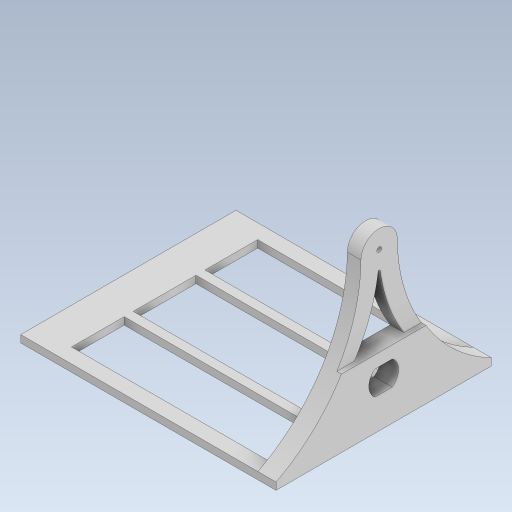
# Autodesk Inventor part: base plate main
Saved by Autodesk Inventor 2023 (Build 270158000, 158)
## iProperties
Created: 2023-03-24
Part Number: base plate main
Material: Generic
Document SubType Name: Modeling
Designer: AggyT
Density: 1 g/cm^3
Appearance: Default
Author: AggyT
Autodesk Inventor part; units mm, degrees
ref_plane "YZ Plane" through (0, 0, 0) normal (1, 0, 0) x (0, 1, 0)
ref_plane "XZ Plane" through (0, 0, 0) normal (0, 1, 0) x (-1, 0, 0)
sketch "Sketch1" plane through (0, 0, 0) normal (0, 1, 0) x (-1, 0, 0)
  line L0 (0, 0) -> (-203.2, 0)
  line L1 (-203.2, 0) -> (-203.2, -177.8)
  line L2 (-203.2, -177.8) -> (0, -177.8)
  line L3 (0, -177.8) -> (0, 0)
  dimension "d0" = 203.2
  dimension "d1" = 177.8
  constraints: 8 end point, 2 parallel, 1 horizontal, 1 perpendicular
  measures "d0" distance of L2.end L1.end
  measures "d1" distance of L1.end L0.end
extrude "Extrusion1" add sketch "Sketch1" along normal blind 10.16
sketch "Sketch2" plane through (0, 10.16, 0) normal (0, 1, 0) x (1, 0, 0)
  line L0 (203.2, 0) -> (203.2, 177.8) projected
  line L1 (203.2, 0) -> (177.8, 0)
  line L2 (177.8, 0) -> (177.8, 177.8)
  line L3 (177.8, 177.8) -> (203.2, 177.8)
  line L4 (203.2, 177.8) -> (203.2, 0)
  point P0 (0, 0)
  dimension "d4" = 25.4
  constraints: 8 end point, 2 parallel, 1 horizontal, 1 perpendicular
  measures "d4" distance of L2.end L3.end
extrude "Extrusion2" add sketch "Sketch2" along normal blind 42.5408
sketch "Sketch3" plane through (177.8, 10.16, -177.8) normal (-1, 0, 0) x (0, 0, 1)
  circle A0 centre (88.9, 25.4) radius 10.3886
  line L0 (81.407, 32.5957) -> (96.393, 32.5957)
  line L1 (81.5172, 18.0912) -> (96.2828, 18.0912)
  line L2 (0, 0) -> (177.8, 0) projected
  line L3 (82.9273, 33.9) -> (94.8727, 33.9)
  line L4 (82.9273, 16.9) -> (94.8727, 16.9)
  point P0 (177.8, -10.16)
  point P1 (88.9, -101.6)
  point P2 (88.8996, -101.6)
  point P3 (100.9466, -114.2832)
  point P4 (102.2534, -114.2832)
  point P5 (114.3004, -101.6)
  point P6 (114.3, -101.6)
  point P7 (159.1068, 0)
  point P8 (88.9, -76.6381)
  point P9 (114.2997, -101.509)
  point P10 (18.6932, 0)
  dimension "d7" = 20.7772
  dimension "d9" = 14.986
  dimension "d45" = 25.4
  dimension "d58" = 8.5
  dimension "d59" = 8.5
  constraints: 8 end point, 2 horizontal, 2 parallel, 10 other
  measures "d9" distance of L0.start L0.end
  measures "d45" distance from line of L2 point (88.9, 25.4)
  measures "d58" distance from line of point (88.9, 25.4) L3
  measures "d59" distance from line of L4 point (88.9, 25.4)
extrude "Extrusion3" cut sketch "Sketch3" against normal blind 50.8 contours A0 L1 L0
sketch "Sketch5" plane through (177.8, 10.16, -177.8) normal (-1, 0, 0) x (0, 0, 1)
  line L0 (-12.7, 203.2) -> (190.5, 203.2)
  line L1 (190.5, 203.2) -> (190.5, 0)
  line L2 (-12.7, 0) -> (-12.7, 203.2)
  line L3 (-12.7, 101.6) -> (190.5, 101.6)
  circle A0 centre (88.9, 101.6) radius 1.5635
  circle A1 centre (88.9, 101.6) radius 12.7
  arc A2 (13.581, 0) -> (76.2003, 101.691) centre (-39.021, 102.5166) ccw
  arc A3 (23.8054, 0) -> (88.9, 95.25) centre (-25.9987, 103.9047) ccw
  line L4 (88.9, -246.9942) -> (88.9, 203.2)
  arc A4 (101.5997, 101.691) -> (164.219, 0) centre (216.821, 102.5166) ccw
  arc A5 (88.9, 95.25) -> (153.9946, 0) centre (203.7987, 103.9047) ccw
  line L5 (153.9946, 0) -> (164.219, 0)
  line L6 (13.581, 0) -> (23.8054, 0)
  line L7 (-12.7, 0) -> (190.5, 0)
  line L8 (177.8, 0) -> (0, 0) projected
  line L9 (177.8, 42.5408) -> (0, 42.5408) projected
  line L10 (88.9, 42.5408) -> (88.9, 0)
  line L11 (0, 0) -> (177.8, 0) projected
  line L12 (13.581, 0) -> (-12.7, 0)
  line L13 (164.219, 0) -> (190.5, 0)
  point P0 (177.8, -10.16)
  point P1 (88.9, -101.6)
  point P2 (88.8996, -101.6)
  point P3 (100.9466, -114.2832)
  point P4 (102.2534, -114.2832)
  point P5 (114.3004, -101.6)
  point P6 (114.3, -101.6)
  point P7 (159.1068, 0)
  point P8 (88.9, -21.8971)
  point P9 (114.2997, -101.509)
  point P10 (88.9, 0)
  point P11 (76.2, 101.6)
  point P12 (76.1996, 101.6)
  point P13 (59.3636, 42.5408)
  point P14 (71.5262, 42.5408)
  point P15 (88.2466, 88.9168)
  point P16 (89.5534, 88.9168)
  point P17 (106.2738, 42.5408)
  point P18 (118.4364, 42.5408)
  point P19 (101.6004, 101.6)
  point P20 (101.6, 101.6)
  dimension "d34" = 25.4
  dimension "d31" = 203.2
  dimension "d32" = 203.2
  dimension "d33" = 3.127
  dimension "d35" = 115.2242
  dimension "d36" = 115.2242
  dimension "d37" = 26.281
  dimension "d38" = 6.35
  dimension "d39" = 101.6
  dimension "d40" = 10.2243
  constraints: 22 end point, 10 midpoint, 8 point on circle, 5 centre point, 5 horizontal, 5 symmetric about line, 1 coincident, 1 parallel, 1 perpendicular, 1 vertical, 6 other
  measures "d31" distance of L1.end L2.start
  measures "d32" distance of L0.end L1.end
  measures "d33" diameter of A0
  measures "d35" radius of A2
  measures "d36" radius of A3
  measures "d37" distance of L2.start L6.start
  measures "d38" distance of point (88.9, 101.6) A3.end
  measures "d39" distance from line of A0.centre L5
  measures "d40" distance of L6.start L6.end
extrude "Extrusion4" add sketch "Sketch5" against normal blind 9.525 contours L4 A0 L3 A1 | A1 L3 A0 L4 | L3 A0 L4 A3 A1 | A1 A3 L9 A2 | A3 L4 A1 | A1 A5 L4 A0 L3 | A4 L9 A5 A1 | L4 A5 A1
sketch "Sketch6" plane through (177.8, 10.16, -177.8) normal (-1, 0, 0) x (0, 0, 1)
  arc A0 (13.581, 0) -> (76.2003, 101.691) centre (-39.021, 102.5166) ccw projected
  arc A1 (101.5997, 101.691) -> (164.219, 0) centre (216.821, 102.5166) ccw projected
  line L0 (177.8, 0) -> (177.8, 42.5408) projected
  line L1 (0, 0) -> (177.8, 0) projected
  line L2 (177.8, 42.5408) -> (0, 42.5408) projected
  line L3 (0, 0) -> (0, 42.5408) projected
  arc A2 (13.581, 0) -> (59.3636, 42.5408) centre (-39.021, 102.5166) ccw
  arc A3 (101.6004, 101.6) -> (118.4364, 42.5408) centre (216.821, 102.5166) ccw projected
  arc A4 (118.4364, 42.5408) -> (164.219, 0) centre (216.821, 102.5166) ccw
  line L4 (0, 42.5408) -> (59.3636, 42.5408) projected
  line L5 (59.3636, 42.5408) -> (0, 42.5408)
  line L6 (0, 42.5408) -> (0, 0)
  line L7 (177.8, 0) -> (0, 0) projected
  line L8 (0, 0) -> (13.581, 0)
  line L9 (164.219, 0) -> (177.8, 0)
  line L10 (177.8, 0) -> (177.8, 42.5408)
  line L11 (118.4364, 42.5408) -> (177.8, 42.5408) projected
  line L12 (118.4364, 42.5408) -> (177.8, 42.5408)
  point P0 (177.8, -10.16)
  point P1 (118.4364, 42.5408)
  point P2 (59.3636, 42.5408)
  constraints: 12 end point, 4 point on circle, 3 concentric, 2 centre point, 2 collinear, 1 perpendicular
extrude "Extrusion5" cut sketch "Sketch6" against normal blind 50.8 contours L1 L3 L2 A0 | A1 L2 L0 L1
sketch "Sketch7" plane through (0, 0, 0) normal (0, -1, 0) x (1, 0, 0)
  line L0 (203.2, 0) -> (203.2, -177.8) projected
  line L1 (0, 0) -> (203.2, 0)
  line L2 (203.2, 0) -> (203.2, -177.8)
  line L3 (203.2, -177.8) -> (0, -177.8)
  line L4 (0, -177.8) -> (0, 0)
  constraints: 8 end point, 2 parallel, 1 horizontal, 1 perpendicular
extrude "Extrusion6" cut sketch "Sketch7" against normal blind 5.08
sketch "Sketch8" plane through (0, 10.16, -177.8) normal (-1, 0, 0) x (0, 0, 1)
  line L0 (0, -5.08) -> (0, 0) projected
  line L1 (0, 0) -> (177.8, 0)
  line L2 (177.8, 0) -> (177.8, -5.08)
  line L3 (177.8, -5.08) -> (0, -5.08)
  line L4 (0, -5.08) -> (0, 0)
  point P0 (177.8, -10.16)
  constraints: 8 end point, 2 parallel, 1 horizontal, 1 perpendicular
extrude "Extrusion7" cut sketch "Sketch8" against normal blind 11.8364
ref_plane "Work Plane1" through (177.8, 10.16, -88.9) normal (0, 0, 1) x (1, 0, 0)
sketch "Sketch9" plane through (0, 5.08, 0) normal (0, -1, 0) x (1, 0, 0)
  line L0 (177.8, -177.8) -> (11.8364, -177.8) projected
  line L1 (203.2, 0) -> (11.8364, 0)
  line L2 (11.8364, 0) -> (11.8364, -177.8)
  line L3 (11.8364, -177.8) -> (203.2, -177.8)
  line L4 (203.2, -177.8) -> (203.2, 0)
  line L5 (177.8, -177.8) -> (203.2, -177.8) projected
  line L6 (180.173, -177.8) -> (180.173, -117.1956)
  line L7 (203.2, -59.3636) -> (203.2, -118.4364) projected
  line L8 (203.2, -117.1956) -> (11.8364, -117.1956)
  line L9 (11.8364, -177.8) -> (11.8364, 0) projected
  line L10 (155.6362, -177.8) -> (155.6362, -164.211)
  line L11 (177.8, -164.219) -> (203.2, -164.219) projected
  line L12 (203.2, -164.219) -> (11.8364, -164.219)
  line L13 (102.4836, -164.219) -> (102.4836, -153.9828)
  line L14 (203.2, 0) -> (203.2, -177.8) projected
  line L15 (203.2, -153.9828) -> (11.8364, -153.9828)
  line L16 (132.8442, -117.1956) -> (132.8442, -110.8456)
  line L17 (203.2, -110.8456) -> (11.8364, -110.8456)
  line L18 (332.5893, -177.8) -> (332.5893, 0)
  line L19 (203.2, -96.2828) -> (203.2, -81.5172) projected
  line L20 (203.2, -88.9) -> (11.8364, -88.9)
  line L21 (203.2, -60.6044) -> (11.8364, -60.6044)
  line L22 (203.2, -13.581) -> (11.8364, -13.581)
  line L23 (203.2, -23.8172) -> (11.8364, -23.8172)
  line L24 (203.2, -66.9544) -> (11.8364, -66.9544)
  line L25 (177.8, 0) -> (177.8, -177.8) projected
  line L26 (177.8, 0) -> (177.8, -177.8)
  line L27 (11.8364, -201.1873) -> (37.2364, -201.1873)
  line L28 (37.2364, -177.8) -> (37.2364, 0)
  line L29 (11.8364, 0) -> (177.8, 0) projected
  point P0 (0, 0)
  point P1 (37.2364, -164.219)
  point P2 (37.2364, -117.1956)
  point P3 (37.2364, -153.9828)
  point P4 (177.8, -153.9828)
  point P5 (177.8, -117.1956)
  point P6 (37.2364, -66.9544)
  point P7 (37.2364, -110.8456)
  point P8 (177.8, -110.8456)
  point P9 (177.8, -66.9544)
  point P10 (37.2364, -23.8172)
  point P11 (37.2364, -60.6044)
  point P12 (177.8, -60.6044)
  point P13 (177.8, -23.8172)
  point P14 (37.2364, 0)
  point P15 (37.2364, -13.581)
  point P16 (177.8, -13.581)
  point P17 (11.8364, -13.581)
  point P18 (11.8364, -164.219)
  point P19 (180.173, -164.219)
  dimension "d51" = 60.6044
  dimension "d52" = 13.589
  dimension "d53" = 10.2362
  dimension "d54" = 6.35
  dimension "d55" = 25.4
  constraints: 42 end point, 13 point on line, 8 symmetric about line, 7 perpendicular, 5 vertical, 2 horizontal, 2 midpoint, 2 parallel
  measures "d51" distance of L6.start L6.end
  measures "d52" distance of L10.start L10.end
  measures "d53" distance of L13.start L13.end
  measures "d54" distance of L16.start L16.end
  measures "d55" distance of L27.start L27.end
extrude "Extrusion8" cut sketch "Sketch9" against normal through all contours L25 L11 L6 L3 | L0 L10 L12 L25 | L0 L28 L12 L10 | L6 L11 L4 L3 | L0 L2 L12 L28 | L15 L28 L8 L25 | L17 L28 L20 L25 | L20 L28 L24 L25 | L21 L28 L23 L25 | L25 L1 L4 L22 | L22 L28 L1 L25 | L22 L2 L1 L28
sketch "Sketch10" plane through (177.8, 111.76, -88.9) normal (-1, 0, 0) x (0, 0, 1)
  arc A0 (7.3828, -83.5088) -> (7.493, -69.0043) centre (0, -76.2) ccw projected
  circle A1 centre (0, -76.2) radius 10.3886
  line L0 (-16.5091, -76.2) -> (-16.5091, -84.7)
  line L1 (-5.9727, -84.7) -> (5.9727, -84.7)
  line L2 (-16.5091, -76.2) -> (-16.5091, -67.7)
  line L3 (-5.9727, -67.7) -> (10.3883, -67.7)
  line L4 (-7.493, -69.0043) -> (7.493, -69.0043) projected
  point P0 (88.9, -111.76)
  point P1 (7.493, -69.0043)
  point P2 (5.9727, -67.7)
  point P3 (7.3828, -83.5088)
  dimension "d62" = 8.5
  dimension "d63" = 8.5
  constraints: 8 end point, 3 point on circle, 1 centre point, 1 coincident, 1 horizontal, 1 parallel, 1 perpendicular, 1 vertical
  measures "d62" distance of L0.start L0.end
  measures "d63" distance of L0.start L2.end
extrude "Extrusion9" cut sketch "Sketch10" against normal through all contours A1 L1 L4 A0 | L4 A1 L3
sketch "Sketch11" plane through (203.2, 52.7008, -59.3636) normal (1, 0, 0) x (0, 0, -1)
  line L0 (-65.6844, 19.5873) -> (128.5678, 19.5873)
  line L1 (128.5678, 19.5873) -> (128.5678, -67.3009)
  line L2 (128.5678, -67.3009) -> (-65.6844, -67.3009)
  line L3 (-65.6844, -67.3009) -> (-65.6844, 19.5873)
  point P0 (-59.3636, -52.7008)
  constraints: 8 end point, 2 parallel, 1 horizontal, 1 perpendicular
extrude "Extrusion10" cut sketch "Sketch11" against normal blind 12.7
body "Solid1"
